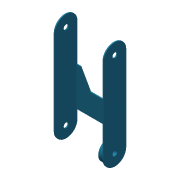
# Autodesk Inventor part: Top_Arm
Saved by Autodesk Inventor 2016 (Build 200138000, 138)
## iProperties
Created: 2015-05-19
Part Number: Top_Arm
Material: Aluminum 6061
Document SubType Name: Modeling
Designer: CHUNGBK
Density: 2.7 g/cm^3
Appearance: Turquoise
Mass: 377.735 g
Surface Area: 866.773 cm^2
Volume: 139.902 cm^3
Author: CHUNGBK
Autodesk Inventor part; units mm, degrees
ref_plane "YZ Plane" through (0, 0, 0) normal (1, 0, 0) x (0, 1, 0)
ref_plane "XZ Plane" through (0, 0, 0) normal (0, 1, 0) x (-1, 0, 0)
sketch "Sketch1" plane through (0, 0, 0) normal (1, 0, 0) x (0, 1, 0)
  circle A0 centre (0, 0) radius 29.3688
  circle A1 centre (220.6625, 0) radius 29.3688
  line L0 (220.6625, -29.3688) -> (0, -29.3688)
  line L1 (220.6625, 29.3687) -> (0, 29.3687)
  line L2 (0, 0) -> (220.6625, 0) construction
  dimension "d0" = 58.7375
  dimension "d1" = 220.6625
  constraints: 6 end point, 4 point on circle, 4 tangent, 2 centre point, 1 coincident, 1 equal radius, 1 horizontal
  measures "d0" distance between parallel lines of L1 L0
  measures "d1" distance of point (0, 0) L2.end
extrude "Extrusion1" add sketch "Sketch1" along normal blind 2.794
ref_plane "Work Plane2" through (64.7065, 0, 0) normal (1, 0, 0) x (0, 0, -1)
ref_plane "Work Plane1" through (126.619, 0, 0) normal (1, 0, 0) x (0, 0, -1)
mirror "Mirror1" about plane through (64.7065, 0, 0) normal (1, 0, 0) of "Extrusion1"
sketch "Sketch2" plane through (2.794, 0, 0) normal (1, 0, 0) x (0, 0, -1)
  line L0 (29.3688, 0) -> (29.3688, 220.6625) projected
  line L1 (29.3688, 123.825) -> (26.5748, 123.825)
  line L2 (26.5748, 123.825) -> (26.5748, 23.8125)
  line L3 (26.5748, 23.8125) -> (29.3688, 23.8125)
  line L4 (29.3688, 23.8125) -> (29.3688, 123.825)
  arc A0 (29.3688, 220.6625) -> (-29.3687, 220.6625) centre (0, 220.6625) ccw projected
  point P0 (0, 0)
  dimension "d6" = 100.0125
  dimension "d7" = 2.794
  dimension "d8" = 96.8375
  constraints: 8 end point, 2 parallel, 1 horizontal, 1 perpendicular, 1 point on line
  measures "d6" distance of L1.end L2.end
  measures "d7" distance of L1.start L1.end
  measures "d8" distance from line of L1 A0.centre
extrude "Extrusion2" add sketch "Sketch2" along normal up to next
sketch "Sketch3" plane through (0, 0, -29.3688) normal (0, 0, -1) x (-1, 0, 0)
  line L0 (0, 0) -> (0, 220.6625) projected
  line L1 (0, 220.6625) -> (-2.794, 220.6625) projected
  line L2 (-2.794, 123.825) -> (-2.794, 220.6625) projected
  line L3 (-2.794, 123.825) -> (-126.619, 123.825) projected
  line L4 (-126.619, 123.825) -> (-126.619, 220.6625) projected
  line L5 (-129.413, 220.6625) -> (-126.619, 220.6625) projected
  line L6 (-129.413, 0) -> (-129.413, 220.6625) projected
  line L7 (-129.413, 0) -> (-126.619, 0) projected
  line L8 (-126.619, 0) -> (-126.619, 23.8125) projected
  line L9 (-2.794, 23.8125) -> (-126.619, 23.8125) projected
  line L10 (-2.794, 0) -> (-2.794, 23.8125) projected
  line L11 (0, 0) -> (-2.794, 0) projected
  line L12 (-116.713, 123.825) -> (-91.694, 79.375)
  line L13 (-91.694, 79.375) -> (-37.719, 79.375)
  line L14 (-37.719, 79.375) -> (-12.7, 123.825)
  line L15 (-64.7065, 79.375) -> (-64.7065, 123.825)
  point P0 (0, 0)
  dimension "d11" = 12.7
  dimension "d12" = 12.7
  dimension "d13" = 53.975
  dimension "d14" = 44.45
  constraints: 8 end point, 2 midpoint, 2 point on line, 1 horizontal, 1 vertical
  measures "d11" distance from line of L12.start L6
  measures "d12" distance from line of L0 L14.end
  measures "d13" distance of L12.end L13.end
  measures "d14" distance between parallel lines of L13 L3
extrude "Extrusion3" cut sketch "Sketch3" against normal blind 2.794 contours L14 L13 L15 L3 | L15 L13 L12 L3
sketch "Sketch5" plane through (126.619, 0, 29.3687) normal (-1, 0, 0) x (0, 0, 1)
  circle A0 centre (-29.3687, 0) radius 25.4
  dimension "d21" = 50.8
  constraints: 1 centre point, 1 coincident
  measures "d21" diameter of A0
extrude "Extrusion5" add sketch "Sketch5" along normal blind 15.24
sketch "Sketch4" plane through (129.413, 0, 29.3687) normal (1, 0, 0) x (0, 0, -1)
  arc A0 (58.7375, 220.6625) -> (0, 220.6625) centre (29.3687, 220.6625) ccw projected
  circle A1 centre (29.3687, 220.6625) radius 6.35
  circle A2 centre (29.3687, 0) radius 6.35
  dimension "d17" = 12.7
  dimension "d18" = 12.7
  constraints: 2 centre point, 2 coincident
  measures "d17" diameter of A1
  measures "d18" diameter of A2
extrude "Extrusion4" cut sketch "Sketch4" against normal through all
body "Solid1"
